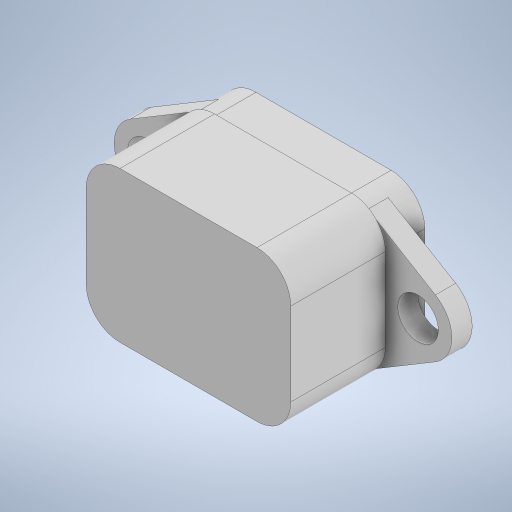
# Autodesk Inventor part: power_socket_24V
Saved by Autodesk Inventor 2023 (Build 270158000, 158)
## iProperties
Created: 2023-06-03
Part Number: power_socket_24V
Material: 一般
Document SubType Name: Modeling
Designer: 310611102
Density: 1 g/cm^3
Appearance: 預設
Author: 310611102
Autodesk Inventor part; units mm, degrees
ref_plane "YZ Plane" through (0, 0, 0) normal (1, 0, 0) x (0, 1, 0)
ref_plane "XZ Plane" through (0, 0, 0) normal (0, 1, 0) x (-1, 0, 0)
ref_plane "XY Plane" through (0, 0, 0) normal (0, 0, 1) x (1, 0, 0)
sketch "Sketch1" plane through (0, 0, 0) normal (0, 0, 1) x (1, 0, 0)
  line L0 (-10, 11) -> (10, 11)
  line L1 (15, 6) -> (15, -6)
  line L2 (10, -11) -> (-10, -11)
  line L3 (-15, -6) -> (-15, 6)
  line L4 (-15, 11) -> (15, -11) construction
  line L5 (15, 11) -> (-15, -11) construction
  arc A0 (-10, 11) -> (-15, 6) centre (-10, 6) ccw
  arc A1 (15, 6) -> (10, 11) centre (10, 6) ccw
  arc A2 (10, -11) -> (15, -6) centre (10, -6) ccw
  arc A3 (-15, -6) -> (-10, -11) centre (-10, -6) ccw
  point P0 (0, 0)
  dimension "d0" = 22
  dimension "d1" = 30
  dimension "d2" = 5
  constraints: 12 end point, 8 point on circle, 8 point on line, 8 tangent, 4 centre point, 3 equal radius, 2 midpoint, 2 parallel, 1 horizontal, 1 perpendicular
  measures "d0" distance of L5.start L4.end
  measures "d1" distance of L4.start L5.start
  measures "d2" radius of A0
extrude "Extrusion1" add sketch "Sketch1" along normal blind 6
sketch "Sketch2" plane through (0, 0, 6) normal (0, 0, 1) x (1, 0, 0)
  arc A0 (-10, 11) -> (-15, 6) centre (-10, 6) ccw projected
  line L0 (-12.5725, 10.2875) -> (-22.5725, 4.2875)
  arc A1 (-22.5725, 4.2875) -> (-22.5725, -4.2875) centre (-20, 0) ccw
  line L1 (-22.5725, -4.2875) -> (-12.5725, -10.2875)
  arc A2 (-15, -6) -> (-10, -11) centre (-10, -6) ccw projected
  line L2 (-15, 6) -> (-15, -6) projected
  line L3 (0, 0) -> (0, 5.4971)
  arc A3 (15, 6) -> (10, 11) centre (10, 6) ccw
  line L4 (12.5725, 10.2875) -> (22.5725, 4.2875)
  arc A4 (22.5725, -4.2875) -> (22.5725, 4.2875) centre (20, 0) ccw
  line L5 (22.5725, -4.2875) -> (12.5725, -10.2875)
  arc A5 (10, -11) -> (15, -6) centre (10, -6) ccw
  line L6 (15, 6) -> (15, -6)
  dimension "d5" = 5
  dimension "d6" = 40
  constraints: 14 point on circle, 12 end point, 11 symmetric about line, 4 centre point, 4 tangent, 1 horizontal alignment, 1 vertical, 3 other
  measures "d5" radius of A1
  measures "d6" distance of A4.centre A1.centre
extrude "Extrusion2" add sketch "Sketch2" against normal blind 3
sketch "Sketch3" plane through (0, 0, 6) normal (0, 0, 1) x (1, 0, 0)
  circle A0 centre (-20, 0) radius 3
  circle A1 centre (20, 0) radius 3
  arc A2 (-22.5725, 4.2875) -> (-22.5725, -4.2875) centre (-20, 0) ccw projected
  arc A3 (22.5725, -4.2875) -> (22.5725, 4.2875) centre (20, 0) ccw projected
  point P0 (0, 0)
  dimension "d9" = 6
  dimension "d10" = 6
  constraints: 2 centre point, 2 concentric
  measures "d9" diameter of A0
  measures "d10" diameter of A1
extrude "Extrusion3" cut sketch "Sketch3" against normal blind 3
sketch "Sketch4" plane through (0, 0, 6) normal (0, 0, 1) x (1, 0, 0)
  line L0 (-10.15, -11.15) -> (10.15, -11.15)
  line L1 (15.15, -6.15) -> (15.15, 6.15)
  line L2 (10.15, 11.15) -> (-10.15, 11.15)
  line L3 (-15.15, 6.15) -> (-15.15, -6.15)
  line L4 (-15.15, -11.15) -> (15.15, 11.15) construction
  line L5 (15.15, -11.15) -> (-15.15, 11.15) construction
  arc A0 (-10.15, 11.15) -> (-15.15, 6.15) centre (-10.15, 6.15) ccw
  arc A1 (15.15, 6.15) -> (10.15, 11.15) centre (10.15, 6.15) ccw
  arc A2 (10.15, -11.15) -> (15.15, -6.15) centre (10.15, -6.15) ccw
  arc A3 (-15.15, -6.15) -> (-10.15, -11.15) centre (-10.15, -6.15) ccw
  point P0 (0, 0)
  dimension "d13" = 22.3
  dimension "d14" = 30.3
  dimension "d15" = 5
  constraints: 12 end point, 8 point on circle, 8 point on line, 8 tangent, 4 centre point, 3 equal radius, 2 midpoint, 2 parallel, 1 horizontal, 1 perpendicular
  measures "d13" distance of L5.start L4.end
  measures "d14" distance of L4.end L5.end
  measures "d15" radius of A0
extrude "Extrusion4" add sketch "Sketch4" along normal blind 14
sketch "Sketch5" plane through (0, 0, 0) normal (0, 0, -1) x (-1, 0, 0)
  line L0 (-7, 8) -> (7, 8)
  line L1 (12, 3) -> (12, -4)
  line L2 (8, -8) -> (-8, -8)
  line L3 (-12, -4) -> (-12, 3)
  line L4 (-12, 8) -> (12, -8) construction
  line L5 (12, 8) -> (-12, -8) construction
  line L6 (-12, 3) -> (-7, 8)
  line L7 (7, 8) -> (12, 3)
  arc A0 (-12, -4) -> (-8, -8) centre (-8, -4) ccw
  arc A1 (8, -8) -> (12, -4) centre (8, -4) ccw
  point P0 (0, 0)
  dimension "d18" = 16
  dimension "d19" = 24
  dimension "d20" = 5
  dimension "d21" = 5
  dimension "d22" = 5
  dimension "d23" = 5
  dimension "d24" = 4
  constraints: 16 end point, 8 point on line, 4 point on circle, 4 tangent, 2 centre point, 2 midpoint, 2 parallel, 1 equal radius, 1 horizontal, 1 perpendicular
  measures "d18" distance of L5.start L4.end
  measures "d19" distance of L4.start L5.start
  measures "d20" distance of L3.end L4.start
  measures "d21" distance of L0.start L4.start
  measures "d22" distance of L0.end L5.start
  measures "d23" distance of L1.start L5.start
  measures "d24" radius of A0
extrude "Extrusion5" cut sketch "Sketch5" against normal blind 17
sketch "Sketch7" plane through (0, 0, 17) normal (0, 0, -1) x (-1, 0, 0)
  line L0 (0.5, 3.8693) -> (-0.5, 3.8693)
  line L1 (-0.5, 3.8693) -> (-0.5, 0.6693)
  line L2 (-0.5, 0.6693) -> (0.5, 0.6693)
  line L3 (0.5, 0.6693) -> (0.5, 3.8693)
  line L4 (0.5, 3.8693) -> (-0.5, 0.6693) construction
  line L5 (-0.5, 3.8693) -> (0.5, 0.6693) construction
  line L6 (3.4545, 0.6693) -> (2.4545, 0.6693)
  line L7 (2.4545, 0.6693) -> (2.4545, -2.5307)
  line L8 (2.4545, -2.5307) -> (3.4545, -2.5307)
  line L9 (3.4545, -2.5307) -> (3.4545, 0.6693)
  line L10 (3.4545, 0.6693) -> (2.4545, -2.5307) construction
  line L11 (2.4545, 0.6693) -> (3.4545, -2.5307) construction
  line L12 (0, 0) -> (0, -2.165)
  line L13 (-3.4545, 0.6693) -> (-2.4545, 0.6693)
  line L14 (-2.4545, 0.6693) -> (-2.4545, -2.5307)
  line L15 (-2.4545, -2.5307) -> (-3.4545, -2.5307)
  line L16 (-3.4545, -2.5307) -> (-3.4545, 0.6693)
  line L17 (-3.4545, 0.6693) -> (-2.4545, -2.5307) construction
  line L18 (-2.4545, 0.6693) -> (-3.4545, -2.5307) construction
  point P0 (0, 2.2693)
  point P1 (2.9545, -0.9307)
  point P2 (-2.9545, -0.9307)
  point P3 (-2.9545, 0.6693)
  dimension "d27" = 1
  dimension "d28" = 1
  dimension "d29" = 3.2
  dimension "d30" = 3.2
  dimension "d31" = 0
  constraints: 38 end point, 5 midpoint, 5 symmetric about line, 4 parallel, 2 horizontal, 2 perpendicular, 1 coincident, 1 vertical
  measures "d27" distance of L0.start L0.end
  measures "d28" distance of L13.start L13.end
  measures "d29" distance of L13.end L14.end
  measures "d30" distance of L2.end L0.start
  measures "d31" distance from line of point (-2.955, 0.669) L2
extrude "Extrusion6" add sketch "Sketch7" along normal blind 14
equation "\"d21\" = d20"
equation "\"d22\" = d20"
equation "\"d23\" = d22"
body "Solid1"
